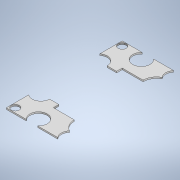
# Autodesk Inventor part: Top Cover Other Side
Saved by Autodesk Inventor 2020 (Build 240168000, 168)
## iProperties
Created: 2019-07-25
Part Number: Top Cover Other Side
Material: Generic
Document SubType Name: Modeling
Designer: Paul
Density: 1 g/cm^3
Appearance: Default
Author: Paul
Autodesk Inventor part; units mm, degrees
ref_plane "YZ Plane" through (0, 0, 0) normal (1, 0, 0) x (0, 1, 0)
ref_plane "XZ Plane" through (0, 0, 0) normal (0, 1, 0) x (-1, 0, 0)
ref_plane "XY Plane" through (0, 0, 0) normal (0, 0, 1) x (1, 0, 0)
sketch "Sketch1" plane through (0, 0, 0) normal (0, 1, 0) x (-1, 0, 0)
  line L0 (16, 16) -> (-16, 16)
  line L1 (-16, 16) -> (-16, -16)
  line L2 (-16, -16) -> (16, -16)
  line L3 (16, -16) -> (16, 16)
  line L4 (16, 16) -> (-16, -16) construction
  line L5 (-16, 16) -> (16, -16) construction
  point P0 (0, 0)
  dimension "d0" = 32
  dimension "d1" = 32
  constraints: 12 end point, 2 midpoint, 2 parallel, 1 horizontal, 1 perpendicular
  measures "d0" distance of L2.end L1.end
  measures "d1" distance of L1.end L0.end
extrude "Extrusion1" add sketch "Sketch1" along normal blind 0.4
sketch "Sketch2" plane through (0, 0.4, 0) normal (0, 1, 0) x (1, 0, 0)
  line L0 (-9.5, -9.5) -> (9.5, -9.5)
  line L1 (9.5, -9.5) -> (9.5, 9.5)
  line L2 (9.5, 9.5) -> (-9.5, 9.5)
  line L3 (-9.5, 9.5) -> (-9.5, -9.5)
  line L4 (-9.5, -9.5) -> (9.5, 9.5) construction
  line L5 (9.5, -9.5) -> (-9.5, 9.5) construction
  circle A0 centre (0, 9.5) radius 3.75
  circle A1 centre (0, -9.5) radius 3.75
  point P0 (0, 0)
  point P1 (-3.75, -9.5)
  point P2 (3.75, -9.5)
  point P3 (3.75, 9.5)
  point P4 (-3.75, 9.5)
  dimension "d4" = 19
  dimension "d5" = 19
  dimension "d6" = 7.5
  dimension "d7" = 7.5
  constraints: 12 end point, 4 midpoint, 2 centre point, 2 parallel, 1 horizontal, 1 perpendicular
  measures "d4" distance of L2.end L1.end
  measures "d5" distance of L1.end L0.end
  measures "d6" diameter of A0
  measures "d7" diameter of A1
extrude "Extrusion2" cut sketch "Sketch2" against normal blind 0.4
sketch "Sketch3" plane through (0, 0.4, 0) normal (0, 1, 0) x (1, 0, 0)
  line L0 (-16, -16) -> (16, -16) projected
  line L1 (16, 16) -> (-16, 16) projected
  line L2 (0, -16) -> (16, -16)
  line L3 (16, -16) -> (16, 16)
  line L4 (16, 16) -> (0, 16)
  line L5 (0, 16) -> (0, -16)
  point P0 (0, 0)
  constraints: 8 end point, 2 parallel, 1 horizontal, 1 midpoint, 1 perpendicular
extrude "Extrusion3" cut sketch "Sketch3" against normal blind 0.4
sketch "Sketch4" plane through (0, 0.4, 0) normal (0, 1, 0) x (1, 0, 0)
  circle A0 centre (-14.76, -14.76) radius 1.11
  circle A1 centre (-14.76, 14.76) radius 1.11
  line L0 (-16, 16) -> (-16, -16) projected
  line L1 (-16, -16) -> (0, -16) projected
  line L2 (0, 16) -> (-16, 16) projected
  circle A2 centre (0, -14.4) radius 2.4
  circle A3 centre (-14.5, 7.96) radius 2.4
  circle A4 centre (-14.5, -7.96) radius 2.4
  circle A5 centre (-8.9, -14.2) radius 2.4
  circle A6 centre (-8.9, 14.2) radius 2.4
  circle A7 centre (0, 14.4) radius 2.4
  line L3 (0, -16) -> (0, -13.25) projected
  line L4 (0, 13.25) -> (0, 16) projected
  point P0 (0, 0)
  point P1 (-7.3125, -16)
  point P2 (-10.4875, -16)
  point P3 (-10.4875, 16)
  point P4 (-7.3125, 16)
  point P5 (-16, -6.0865)
  point P6 (-16, -9.8335)
  point P7 (-16, 9.8335)
  point P8 (-16, 6.0865)
  dimension "d12" = 2.22
  dimension "d13" = 2.22
  dimension "d14" = 1.24
  dimension "d15" = 1.24
  dimension "d16" = 1.24
  dimension "d17" = 1.24
  dimension "d18" = 4.8
  dimension "d19" = 4.8
  dimension "d20" = 4.8
  dimension "d21" = 4.8
  dimension "d22" = 4.8
  dimension "d23" = 4.8
  dimension "d24" = 0
  dimension "d26" = 0
  dimension "d28" = 7.1
  dimension "d29" = 1.8
  dimension "d30" = 1.8
  dimension "d31" = 7.1
  dimension "d32" = 1.6
  dimension "d33" = 1.6
  dimension "d34" = 1.5
  dimension "d35" = 8.04
  dimension "d36" = 8.04
  dimension "d37" = 1.5
  constraints: 8 centre point
  measures "d12" diameter of A0
  measures "d13" diameter of A1
  measures "d14" distance from line of L0 A0.centre
  measures "d15" distance from line of L1 A0.centre
  measures "d16" distance from line of L2 A1.centre
  measures "d17" distance from line of L0 A1.centre
  measures "d18" diameter of A2
  measures "d19" diameter of A3
  measures "d20" diameter of A4
  measures "d21" diameter of A5
  measures "d22" diameter of A6
  measures "d23" diameter of A7
  measures "d24" distance from line of L3 A2.centre
  measures "d26" distance from line of L4 A7.centre
  measures "d28" distance from line of L0 A6.centre
  measures "d29" distance from line of L2 A6.centre
  measures "d30" distance from line of L1 A5.centre
  measures "d31" distance from line of L0 A5.centre
  measures "d32" distance from line of A7.centre L2
  measures "d33" distance from line of L1 A2.centre
  measures "d34" distance from line of L0 A3.centre
  measures "d35" distance from line of L2 A3.centre
  measures "d36" distance from line of L1 A4.centre
  measures "d37" distance from line of L0 A4.centre
extrude "Extrusion4" cut sketch "Sketch4" against normal blind 0.4 contours A0 | A1 | A2 | A5 L1 | A4 L0 | A3 L0 | A7 | L2 A6 picked at (-8.777, -14.4925) picked at (-14.5551, -7.8666) picked at (-14.7976, 7.5771) picked at (-8.6453, 14.6416)
sketch "Sketch5" plane through (0, 0.4, 0) normal (0, 1, 0) x (1, 0, 0)
  line L0 (-9.5, -9.5) -> (-9.5, 9.5) projected
  line L1 (-16, -7.96) -> (-9.5, -7.96)
  line L2 (-9.5, -7.96) -> (-9.5, 7.96)
  line L3 (-9.5, 7.96) -> (-16, 7.96)
  line L4 (-16, 7.96) -> (-16, -7.96)
  point P0 (0, 0)
  dimension "d40" = 15.92
  constraints: 8 end point, 2 parallel, 1 horizontal, 1 perpendicular, 1 point on line
  measures "d40" distance between parallel lines of L1 L3
extrude "Extrusion5" cut sketch "Sketch5" against normal blind 0.4
body "Solid1"
